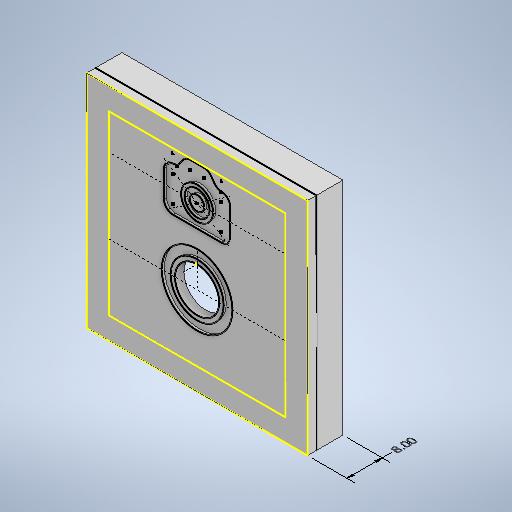
# Autodesk Inventor part: Tapa_camara
Saved by Autodesk Inventor 2025.1 (Build 291241000, 241)
## iProperties
Created: 2025-11-25
Part Number: Tapa_camara
Material: Genérico
Document SubType Name: Modeling
Designer: Diego
Density: 1 g/cm^3
Appearance: Valor por defecto
Author: Diego
Autodesk Inventor part; units mm, degrees
ref_plane "YZ Plane" through (0, 0, 0) normal (1, 0, 0) x (0, 1, 0)
ref_plane "XZ Plane" through (0, 0, 0) normal (0, 1, 0) x (-1, 0, 0)
ref_plane "XY Plane" through (0, 0, 0) normal (0, 0, 1) x (1, 0, 0)
sketch "Boceto1" plane through (0, 0, 0) normal (0, 0, 1) x (1, 0, 0)
  line L0 (-20, -20) -> (20, -20)
  line L1 (20, -20) -> (20, 20)
  line L2 (20, 20) -> (-20, 20)
  line L3 (-20, 20) -> (-20, -20)
  line L4 (-20, -20) -> (20, 20) construction
  line L5 (20, -20) -> (-20, 20) construction
  line L6 (-25, 25) -> (25, 25)
  line L7 (25, 25) -> (25, -25)
  line L8 (25, -25) -> (-25, -25)
  line L9 (-25, -25) -> (-25, 25)
  point P0 (0, 0)
  dimension "d0" = 40
  dimension "d1" = 40
  dimension "d2" = 5
  constraints: 20 end point, 4 parallel, 2 midpoint, 2 perpendicular, 1 horizontal, 3 other
  measures "d0" distance of L2.end L1.end
  measures "d1" distance of L1.end L0.end
  measures "d2" distance between parallel lines of L2 L6
extrude "Extrusión1" add sketch "Boceto1" against normal blind 6
extrude "Extrusión2" add sketch "Boceto1" along normal blind 2 contours L3 L2 L1 L0 | L6 L7 L8 L9
sketch "Boceto3" plane through (0, 0, 2) normal (0, 0, 1) x (1, 0, 0)
  line L0 (25, -25) -> (-25, -25) projected
  line L1 (-25, -25) -> (-25, 25) projected
  line L2 (-25, 25) -> (25, 25) projected
  line L3 (25, 25) -> (25, -25) projected
  line L4 (20, -20) -> (-20, -20) projected
  line L5 (-20, -20) -> (-20, 20) projected
  line L6 (-20, 20) -> (20, 20) projected
  line L7 (20, 20) -> (20, -20) projected
  line L8 (-20, -5) -> (20, -5) construction
  circle A0 centre (0, -5) radius 5
  circle A1 centre (0, -5) radius 6
  circle A2 centre (0, -5) radius 8
  line L9 (-20, 12) -> (20, 12) construction
  line L10 (0, 3) -> (0, -5) construction
  line L11 (5.5, 7) -> (-5.5, 7)
  line L12 (-7.5, 9) -> (-7.5, 15)
  line L13 (7.5, 15) -> (7.5, 9)
  line L14 (7.5, 7) -> (-7.5, 17) construction
  line L15 (-7.5, 7) -> (7.5, 17) construction
  line L16 (-3.9028, 17.8528) -> (-3.2066, 18.8472)
  line L17 (3.2066, 18.8472) -> (3.9028, 17.8528)
  line L18 (-1.5683, 19.7) -> (1.5683, 19.7)
  circle A3 centre (0, 12) radius 1.6258
  circle A4 centre (0, 12) radius 2.8258
  circle A5 centre (0, 12) radius 3.6258
  line L19 (-5.5, 17) -> (-5.5411, 17)
  line L20 (5.5411, 17) -> (5.5, 17)
  arc A6 (-5.5411, 17) -> (-3.9028, 17.8528) centre (-5.5411, 19) ccw
  arc A7 (-1.5683, 19.7) -> (-3.2066, 18.8472) centre (-1.5683, 17.7) ccw
  arc A8 (3.2066, 18.8472) -> (1.5683, 19.7) centre (1.5683, 17.7) ccw
  arc A9 (3.9028, 17.8528) -> (5.5411, 17) centre (5.5411, 19) ccw
  arc A10 (-5.5, 17) -> (-7.5, 15) centre (-5.5, 15) ccw
  arc A11 (-7.5, 9) -> (-5.5, 7) centre (-5.5, 9) ccw
  arc A12 (5.5, 7) -> (7.5, 9) centre (5.5, 9) ccw
  arc A13 (7.5, 15) -> (5.5, 17) centre (5.5, 15) ccw
  point P0 (0, 0)
  point P1 (-4.5, 17)
  point P2 (5.5206, 17)
  dimension "d13" = 15
  dimension "d14" = 10
  dimension "d17" = 1
  dimension "d18" = 2
  dimension "d21" = 9
  dimension "d22" = 15
  dimension "d23" = 10
  dimension "d25" = 3
  dimension "d27" = 3.2517
  dimension "d28" = 1.2
  dimension "d29" = 0.8
  dimension "d30" = 2.7
  dimension "d31" = 125
  dimension "d32" = 2
  dimension "d33" = 2
  constraints: 26 end point, 16 point on circle, 16 tangent, 14 point on line, 13 centre point, 6 equal radius, 5 midpoint, 3 parallel, 3 perpendicular, 2 horizontal, 1 coincident, 1 vertical, 1 vertical alignment, 3 other
  measures "d13" distance between parallel lines of L4 L8
  measures "d14" diameter of A0
  measures "d17" radial gap between concentric circles of A0 A1
  measures "d21" distance from line of L10.start L9
  measures "d22" distance of L14.end L15.end
  measures "d23" distance of L15.start L14.end
  measures "d25" distance of L14.end point (-4.5, 17)
  measures "d27" diameter of A3
  measures "d28" radial gap between concentric circles of A3 A4
  measures "d29" radial gap between concentric circles of A4 A5
  measures "d30" distance from line of point (5.521, 17) L18
  measures "d31" angle of L19 L16
  measures "d32" radius of A6
  measures "d33" radius of A10
extrude "Extrusión4" cut sketch "Boceto3" against normal through all contours A0
extrude "Extrusión5" cut sketch "Boceto3" against normal blind 0.6 contours A2
extrude "Extrusión6" cut sketch "Boceto3" against normal blind 0.6 contours L11 A11 L12 A10 L19 A6 L16 A7 L18 A8 L17 A9 L20 A13 L13 A12 | A4
sketch "Boceto4" plane through (0, 0, -6) normal (0, 0, -1) x (-1, 0, 0)
  point P0 (0, 0)
equation "\"d1\" = d0"
equation "\"d14\" = D_camara"
equation "\"D_camara\" = 10"
